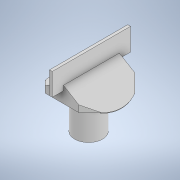
# Autodesk Inventor part: Base_rotativa
Saved by Autodesk Inventor 2021 (Build 250183000, 183)
## iProperties
Created: 2022-01-26
Part Number: Base_rotativa
Material: Genérico
Document SubType Name: Modeling
Designer: pc
Density: 1 g/cm^3
Appearance: Valor por defecto
Author: pc
Autodesk Inventor part; units mm, degrees
ref_plane "YZ Plane" through (0, 0, 0) normal (1, 0, 0) x (0, 1, 0)
ref_plane "XZ Plane" through (0, 0, 0) normal (0, 1, 0) x (-1, 0, 0)
ref_plane "XY Plane" through (0, 0, 0) normal (0, 0, 1) x (1, 0, 0)
sketch "Boceto1" plane through (0, 0, 0) normal (0, 0, 1) x (1, 0, 0)
  line L0 (0, 0) -> (-500, 0)
  line L1 (0, 0) -> (500, 0)
  line L2 (0, 0) -> (0, 300)
  line L3 (-500, 0) -> (0, 300)
  line L4 (500, 0) -> (0, 300)
  dimension "d0" = 500
  dimension "d1" = 500
  dimension "d2" = 300
  constraints: 10 end point, 2 horizontal, 1 perpendicular
  measures "d0" distance of L0.start L0.end
  measures "d1" distance of L0.start L1.end
  measures "d2" distance of L0.start L2.end
extrude "Extrusión1" add sketch "Boceto1" along normal blind 1000
sketch "Boceto2" plane through (-500, 0, 0) normal (0, -1, 0) x (1, 0, 0)
  line L0 (0, 1000) -> (1000, 1000) projected
  line L1 (0, 1000) -> (0, 800)
  line L2 (0, 0) -> (0, 1000) projected
  line L3 (0, 800) -> (200, 1000)
  line L4 (200, 1000) -> (0, 1000)
  line L5 (1000, 1000) -> (800, 1000)
  line L6 (800, 1000) -> (1000, 800)
  line L7 (1000, 0) -> (1000, 1000) projected
  line L8 (1000, 800) -> (1000, 1000)
  line L9 (0, 0) -> (1000, 0) projected
  line L10 (0, 0) -> (0, 200)
  line L11 (200, 0) -> (0, 0)
  line L12 (200, 0) -> (0, 200)
  line L13 (1000, 0) -> (800, 0)
  line L14 (800, 0) -> (1000, 0)
  line L15 (1000, 200) -> (800, 0)
  point P0 (500, 0)
  dimension "d5" = 200
  dimension "d6" = 45
  dimension "d7" = 200
  dimension "d8" = 45
  constraints: 24 end point, 6 point on line, 3 perpendicular, 2 collinear
  measures "d5" distance of L0.start L1.end
  measures "d6" angle of L3 L1
  measures "d7" distance of L0.end L5.end
  measures "d8" angle of L6 L5
extrude "Extrusión2" cut sketch "Boceto2" against normal blind 1000 contours L0 L3 L1 | L0 L7 L6 | L12 L9 L2 | L7 L9 L15
sketch "Boceto3" plane through (0, 300, 1000) normal (0.5144958, 0.8574929, 0) x (0.8574929, -0.5144958, 0)
  line L0 (583.0952, 800) -> (583.0952, 200) projected
  arc A0 (583.0952, 200) -> (583.0952, 800) centre (63.4799, 500) ccw
  line L1 (583.0952, 800) -> (473.0952, 800)
  line L2 (473.0952, 800) -> (473.0952, 200)
  line L3 (473.0952, 200) -> (583.0952, 200)
  line L4 (583.0952, 200) -> (583.0952, 800)
  point P0 (154.3487, 1000)
  dimension "d11" = 600
  dimension "d12" = 110
  constraints: 8 end point, 2 parallel, 2 point on circle, 1 centre point, 1 horizontal, 1 perpendicular
  measures "d11" radius of A0
  measures "d12" distance of L3.end L2.end
extrude "Extrusión3" add sketch "Boceto3" against normal blind 20
sketch "Boceto4" plane through (0, 300, 1000) normal (-0.5144958, 0.8574929, 0) x (0.8574929, 0.5144958, 0)
  line L0 (-583.0952, 800) -> (-583.0952, 200) projected
  arc A0 (-583.0952, 800) -> (-583.0952, 200) centre (-63.4799, 500) ccw
  line L1 (-583.0952, 800) -> (-473.0952, 800)
  line L2 (-473.0952, 800) -> (-473.0952, 200)
  line L3 (-473.0952, 200) -> (-583.0952, 200)
  line L4 (-583.0952, 200) -> (-583.0952, 800)
  point P0 (-154.3487, 1000)
  dimension "d15" = 600
  dimension "d16" = 110
  constraints: 8 end point, 2 parallel, 2 point on circle, 1 centre point, 1 horizontal, 1 perpendicular
  measures "d15" radius of A0
  measures "d16" distance of L2.end L3.end
extrude "Extrusión4" add sketch "Boceto4" against normal blind 20
sketch "Boceto5" plane through (0, 0, 0) normal (0, 0, -1) x (-1, 0, 0)
  line L0 (-300, 120) -> (0, 300) projected
  line L1 (0, 300) -> (0, 200)
  line L2 (0, 200) -> (25, 200)
  line L3 (0, 200) -> (-25, 200)
  line L4 (-25, 200) -> (-25, 600)
  line L5 (-25, 600) -> (25, 600)
  line L6 (25, 600) -> (25, 200)
  point P0 (0, 0)
  dimension "d19" = 100
  dimension "d20" = 25
  dimension "d21" = 25
  dimension "d22" = 400
  constraints: 12 end point, 3 perpendicular, 1 horizontal, 1 parallel, 1 vertical
  measures "d19" distance of L0.end L1.end
  measures "d20" distance of L1.end L2.end
  measures "d21" distance of L1.end L3.end
  measures "d22" distance of L3.end L4.end
extrude "Extrusión5" add sketch "Boceto5" along normal blind 200 and the other way blind 1200
sketch "Boceto6" plane through (-300, 0, 0) normal (0, -1, 0) x (1, 0, 0)
  line L0 (275, 1000) -> (275, 0) projected
  circle A0 centre (275, 500) radius 250
  point P0 (300, 0)
  dimension "d27" = 500
  constraints: 1 centre point, 1 midpoint
  measures "d27" diameter of A0
extrude "Extrusión6" add sketch "Boceto6" along normal blind 700
